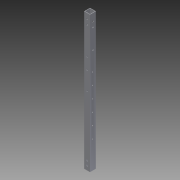
# Autodesk Inventor part: Rebuild Edge Mount 2
Saved by Autodesk Inventor 2014 SP1 (Build 180222100, 222)
## iProperties
Created: 2013-01-21
Part Number: Rebuild Edge Mount 2
Material: Aluminum 6061
Document SubType Name: Modeling
Designer: actoennies
Density: 2.71 g/cm^3
Mass: 240.492 g
Surface Area: 1130.79 cm^2
Volume: 88.7426 cm^3
Appearance: Aluminum - Flat
Author: actoennies
Autodesk Inventor part; units mm, degrees
ref_plane "YZ Plane" through (0, 0, 0) normal (1, 0, 0) x (0, 1, 0)
ref_plane "XZ Plane" through (0, 0, 0) normal (0, 1, 0) x (-1, 0, 0)
ref_plane "XY Plane" through (0, 0, 0) normal (0, 0, 1) x (1, 0, 0)
sketch "Sketch1" plane through (0, 0, 0) normal (0, 1, 0) x (-1, 0, 0)
  line L0 (0, 0) -> (-25.4, 0)
  line L1 (-25.4, 0) -> (-25.4, 25.4)
  line L2 (-25.4, 25.4) -> (0, 25.4)
  line L3 (0, 25.4) -> (0, 0)
  line L4 (-1.5875, 23.8125) -> (-23.8125, 23.8125)
  line L5 (-23.8125, 23.8125) -> (-23.8125, 1.5875)
  line L6 (-23.8125, 1.5875) -> (-1.5875, 1.5875)
  line L7 (-1.5875, 1.5875) -> (-1.5875, 23.8125)
  dimension "d0" = 25.4
  dimension "d2" = 25.4
  dimension "d3" = 1.5875
  constraints: 16 end point, 4 parallel, 2 perpendicular, 1 horizontal, 3 other
  measures "d0" distance of L0.end L1.end
  measures "d2" distance of L1.end L2.end
  measures "d3" distance between parallel lines of L2 L4
extrude "Extrusion1" add sketch "Sketch1" along normal blind 596.9
sketch "Sketch8" plane through (25.4, 0, 25.4) normal (1, 0, 0) x (0, 0, -1)
  circle A0 centre (12.7, 457.2) radius 3.3782
  circle A1 centre (11.1125, 374.65) radius 2.54
  circle A2 centre (11.1125, 323.85) radius 2.54
  circle A3 centre (11.1125, 273.05) radius 2.54
  circle A4 centre (11.1125, 222.25) radius 2.54
  circle A5 centre (11.1125, 171.45) radius 2.54
  circle A6 centre (11.1125, 120.65) radius 2.54
  circle A7 centre (12.7, 565.15) radius 3.3782
  circle A8 centre (12.7, 542.925) radius 3.3782
  line L0 (25.4, 0) -> (0, 0)
  line L1 (0, 596.9) -> (25.4, 596.9)
  line L2 (12.7, 596.9) -> (12.7, 0) construction
extrude "Extrusion7" cut sketch "Sketch8" against normal blind 25.4
sketch "Sketch9" plane through (25.4, 0, 0) normal (0, 0, -1) x (-1, 0, 0)
  circle A0 centre (12.7, 431.8) radius 3.3782 projected
  line L0 (25.4, 440.055) -> (0, 440.055) projected
  line L1 (0, 368.3) -> (0, 440.055) projected
  line L2 (25.4, 368.3) -> (0, 368.3) projected
  line L3 (25.4, 440.055) -> (25.4, 368.3) projected
  circle A1 centre (12.7, 431.8) radius 3.3782 projected
  circle A2 centre (12.7, 381) radius 3.3782 projected
  circle A3 centre (12.7, 19.05) radius 3.302 projected
  circle A4 centre (12.7, 38.1) radius 3.302 projected
  arc A5 (3.175, 50.8) -> (0, 47.625) centre (3.175, 47.625) ccw projected
  line L4 (3.175, 50.8) -> (22.225, 50.8) projected
  arc A6 (25.4, 47.625) -> (22.225, 50.8) centre (22.225, 47.625) ccw projected
  line L5 (25.4, 47.625) -> (25.4, 4.445) projected
  line L6 (25.4, 4.445) -> (0, 4.445) projected
  line L7 (0, 47.625) -> (0, 4.445) projected
  circle A7 centre (12.7, 552.45) radius 3.3782 projected
  circle A8 centre (12.7, 574.675) radius 3.3782 projected
  circle A9 centre (12.7, 301.625) radius 3.3782 projected
extrude "Extrusion8" cut sketch "Sketch9" against normal blind 25.4 contours A0 | A2 | A3 | A4 | A7 | A8 | A9
body "Solid1"
